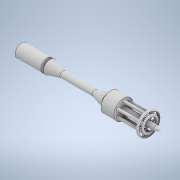
# Autodesk Inventor part: Weapon-Electric-Barrel
Saved by Autodesk Inventor 2020 (Build 240168000, 168)
## iProperties
Created: 2019-11-13
Part Number: Weapon-Electric-Barrel
Material: Generic
Document SubType Name: Modeling
Designer: vifly_01
Density: 1 g/cm^3
Appearance: Default
Author: vifly_01
Autodesk Inventor part; units mm, degrees
ref_plane "YZ Plane" through (0, 0, 0) normal (1, 0, 0) x (0, 1, 0)
ref_plane "XZ Plane" through (0, 0, 0) normal (0, 1, 0) x (-1, 0, 0)
ref_plane "XY Plane" through (0, 0, 0) normal (0, 0, 1) x (1, 0, 0)
sketch "Sketch1" plane through (0, 0, 0) normal (0, 0, 1) x (1, 0, 0)
  circle A0 centre (0, 0) radius 2.5
  dimension "d0" = 5
  constraints: 1 centre point, 1 coincident
  measures "d0" diameter of A0
extrude "Extrusion1" add sketch "Sketch1" along normal blind 10
sketch "Sketch2" plane through (0, 0, 10) normal (0, 0, 1) x (1, 0, 0)
  circle A0 centre (0, 0) radius 1
  dimension "d3" = 2
  constraints: 1 centre point, 1 coincident
  measures "d3" diameter of A0
extrude "Extrusion2" add sketch "Sketch2" along normal blind 1
sketch "Sketch3" plane through (0, 0, 0) normal (0, 0, -1) x (-1, 0, 0)
  circle A0 centre (0, 0) radius 1
  constraints: 1 centre point, 1 coincident
extrude "Extrusion3" add sketch "Sketch3" along normal blind 1
sketch "Sketch4" plane through (0, 0, -1) normal (0, 0, -1) x (-1, 0, 0)
  circle A0 centre (0, 0) radius 2.5
  constraints: 1 centre point, 1 coincident
extrude "Extrusion4" add sketch "Sketch4" along normal blind 5 draft -15
sketch "Sketch5" plane through (0, 0, -6) normal (0, 0, -1) x (-1, 0, 0)
  circle A0 centre (0, 0) radius 1.1603
  constraints: 1 centre point, 1 coincident
extrude "Extrusion5" add sketch "Sketch5" along normal blind 12.5
sketch "Sketch6" plane through (0, 0, -18.5) normal (0, 0, -1) x (-1, 0, 0)
  circle A0 centre (0, 0) radius 1.1603 projected
  circle A1 centre (0, 0) radius 1.1603
  constraints: 1 centre point, 1 coincident
extrude "Extrusion6" add sketch "Sketch6" along normal blind 5 draft 15
sketch "Sketch7" plane through (0, 0, -23.5) normal (0, 0, -1) x (-1, 0, 0)
  circle A0 centre (0, 0) radius 1 projected
  circle A1 centre (0, 0) radius 1
  constraints: 1 centre point, 1 coincident
extrude "Extrusion7" add sketch "Sketch7" along normal blind 1
sketch "Sketch8" plane through (0, 0, -24.5) normal (0, 0, -1) x (-1, 0, 0)
  circle A0 centre (0, 0) radius 3.75
  dimension "d16" = 7.5
  constraints: 1 centre point, 1 coincident
  measures "d16" diameter of A0
extrude "Extrusion8" add sketch "Sketch8" along normal blind 5
sketch "Sketch9" plane through (0, 0, -29.5) normal (0, 0, -1) x (-1, 0, 0)
  circle A0 centre (0, 2.75) radius 0.5
  circle A1 centre (-2.3816, 1.375) radius 0.5
  circle A2 centre (-2.3816, -1.375) radius 0.5
  circle A3 centre (0, -2.75) radius 0.5
  circle A4 centre (2.3816, -1.375) radius 0.5
  circle A5 centre (2.3816, 1.375) radius 0.5
  point P0 (0, 0)
  dimension "d19" = 1
  dimension "d22" = 360
  constraints: 6 centre point, 13 other
  measures "d19" diameter of A0
extrude "Extrusion9" add sketch "Sketch9" along normal blind 10
sketch "Sketch10" plane through (0, 0, -29.5) normal (0, 0, -1) x (-1, 0, 0)
  circle A0 centre (0, 0) radius 1
  constraints: 1 centre point, 1 coincident
extrude "Extrusion10" add sketch "Sketch10" along normal blind 12.5
sketch "Sketch11" plane through (0, 0, -42) normal (0, 0, -1) x (-1, 0, 0)
  circle A0 centre (0, 0) radius 1
  constraints: 1 centre point, 1 coincident
extrude "Extrusion11" add sketch "Sketch11" along normal blind 2 draft -26
sketch "Sketch13" plane through (0, 0, 0) normal (1, 0, 0) x (0, 1, 0)
  arc A0 (4, -39.5001) -> (4, -38.4999) centre (4, -39) ccw
  line L0 (4, -38.4999) -> (4, -39.5001)
  line L1 (0, -55) -> (0, 22) projected
  point P0 (0, 0)
  constraints: 2 end point, 2 point on circle, 1 centre point, 1 vertical
revolve "Revolution2" add sketch "Sketch13" angle 360 about axis through (0, 0, -10) along (0, 0, 1)
ref_plane "Work Plane1" through (0, 0, -27) normal (0, 0, -1) x (-1, 0, 0)
sketch "Sketch15" plane through (0, 0, 0) normal (0, 1, 0) x (-1, 0, 0)
  line L0 (-4, -38.75) -> (-1, -38.75)
  line L1 (-4, -39.25) -> (-1, -39.25)
  line L2 (-1, -29.5) -> (-1, -42) projected
  line L3 (-1, -38.75) -> (-0.75, -38.75)
  line L4 (-1, -39.25) -> (-0.75, -39.25)
  line L5 (-0.75, -39.25) -> (-0.75, -38.75)
  line L6 (-4, -39.25) -> (-4.1, -39.25)
  line L7 (-4.1, -39.25) -> (-4.1, -38.75)
  line L8 (-4.1, -38.75) -> (-4, -38.75)
  point P0 (0, 0)
  dimension "d35" = 0.5
  dimension "d37" = 0.25
  dimension "d38" = 0.1
  constraints: 16 end point, 2 horizontal, 2 perpendicular, 2 point on line, 1 collinear
  measures "d35" distance between parallel lines of L1 L0
  measures "d37" distance of L0.end L3.end
  measures "d38" distance of L1.start L6.end
extrude "Extrusion12" add sketch "Sketch15" along normal mid plane 0.25
pattern_circular "Circular Pattern1" count 6 over 360 about axis through (0, 0, -29.5) along (0, 0, -1) of "Extrusion12"
sketch "Sketch17" plane through (0, 0, 0) normal (1, 0, 0) x (0, 1, 0)
  line L0 (2.25, -39.5) -> (3.25, -39.5) projected
  arc A0 (2.25, -39.5) -> (3.25, -39.5) centre (2.75, -39.5) ccw
  line L1 (3.25, -39.5) -> (2.25, -39.5)
  line L2 (0, -55) -> (0, 22) projected
  point P0 (0, 0)
  constraints: 2 end point, 2 point on circle, 1 centre point, 1 collinear, 1 midpoint
revolve "Revolution3" add sketch "Sketch17" angle 360 about axis through (0, 0, -10) along (0, 0, 1)
body "Solid1"
